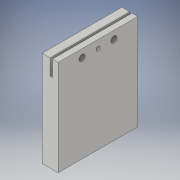
# Autodesk Inventor part: mask holder
Saved by Autodesk Inventor 2017 (Build 210142000, 142)
## iProperties
Created: 2016-12-03
Part Number: mask holder
Material: Generic
Document SubType Name: Modeling
Designer: Darien Morrow
Density: 1 g/cm^3
Appearance: Default
Author: Darien Morrow
Autodesk Inventor part; units mm, degrees
ref_plane "YZ Plane" through (0, 0, 0) normal (1, 0, 0) x (0, 1, 0)
ref_plane "XZ Plane" through (0, 0, 0) normal (0, 1, 0) x (-1, 0, 0)
ref_plane "XY Plane" through (0, 0, 0) normal (0, 0, 1) x (1, 0, 0)
sketch "Sketch1" plane through (0, 0, 0) normal (0, 0, 1) x (1, 0, 0)
  line L0 (-6.35, -38.1) -> (6.35, -38.1)
  line L1 (6.35, -38.1) -> (6.35, 38.1)
  line L2 (6.35, 38.1) -> (-6.35, 38.1)
  line L3 (-6.35, 38.1) -> (-6.35, -38.1)
  line L4 (-6.35, -38.1) -> (6.35, 38.1) construction
  line L5 (6.35, -38.1) -> (-6.35, 38.1) construction
  line L6 (-0.889, 50.8) -> (0.889, 50.8)
  line L7 (0.889, 50.8) -> (0.889, 25.4)
  line L8 (0.889, 25.4) -> (-0.889, 25.4)
  line L9 (-0.889, 25.4) -> (-0.889, 50.8)
  line L10 (-0.889, 50.8) -> (0.889, 25.4) construction
  line L11 (0.889, 50.8) -> (-0.889, 25.4) construction
  point P0 (0, 0)
  point P1 (0, 38.1)
  dimension "d0" = 12.7
  dimension "d1" = 76.2
  dimension "d2" = 1.778
  dimension "d3" = 12.7
  constraints: 24 end point, 5 midpoint, 4 parallel, 2 horizontal, 2 perpendicular
  measures "d0" distance of L2.end L1.end
  measures "d1" distance between parallel lines of L0 L2
  measures "d2" distance of L7.end L8.end
  measures "d3" distance from line of L8 point (0, 38.1)
extrude "Extrusion1" add sketch "Sketch1" along normal blind 63.5 contours L3 L2 L9 L8 L7 L1 L0 | L2 L7 L8 L9
sketch "Sketch2" plane through (0, 0, 0) normal (0, 0, -1) x (-1, 0, 0)
  line L0 (-6.35, 38.1) -> (6.35, 38.1) projected
  line L1 (0, 38.1) -> (-1.778, 38.1)
  line L2 (-1.778, 38.1) -> (-1.778, 25.4)
  line L3 (-1.778, 25.4) -> (0, 25.4)
  line L4 (0, 25.4) -> (0, 38.1)
  point P0 (0, 0)
  dimension "d6" = 1.778
  dimension "d7" = 12.7
  constraints: 8 end point, 2 parallel, 1 horizontal, 1 midpoint, 1 perpendicular
  measures "d6" distance of L3.end L2.end
  measures "d7" distance between parallel lines of L3 L0
extrude "Extrusion2" cut sketch "Sketch2" against normal blind 63.5
sketch "Sketch3" plane through (6.35, -38.1, 0) normal (1, 0, 0) x (0, 0, -1)
  line L0 (0, 76.2) -> (-63.5, 76.2) projected
  line L1 (-63.5, 0) -> (-63.5, 76.2) projected
  point P0 (0, 38.1)
  point P1 (-31.75, 69.85)
  dimension "d10" = 6.35
  dimension "d11" = 31.75
  measures "d10" distance from line of point (-31.75, 69.85) L0
  measures "d11" distance from line of point (-31.75, 69.85) L1
hole "Hole1" at (6.35, 31.75, 31.75) direction (-1, 0, 0) diameter 3.175 end through all
sketch "Sketch4" plane through (6.35, -38.1, 0) normal (1, 0, 0) x (0, 0, -1)
  line L0 (-44.45, 69.8514) -> (-19.05, 69.8514)
  line L1 (0, 0) -> (0, 76.2) projected
  point P0 (0, 38.1)
  dimension "d19" = 25.4
  dimension "d20" = 19.05
  constraints: 2 coincident, 2 end point, 1 horizontal
  measures "d19" distance of L0.start L0.end
  measures "d20" distance from line of L1 L0.end
hole "Hole2" at (6.35, 31.7514, 44.45) at (6.35, 31.7514, 19.05) direction (-1, 0, 0) diameter 4.9784 depth 19.05 tip angle 118 thread size "1/4-20 UNC" class "2B" standard "ANSI Unified Screw Threads"
sketch "Sketch5" plane through (-6.35, -38.1, 0) normal (0, -1, 0) x (1, 0, 0)
  line L0 (6.35, 63.5) -> (6.35, 0) projected
  line L1 (6.35, 57.15) -> (6.35, 6.35)
  dimension "d28" = 50.8
  dimension "d29" = 6.35
  constraints: 2 coincident, 2 end point, 2 point on line
  measures "d28" distance of L1.start L1.end
  measures "d29" distance of L0.start L1.start
hole "Hole3" at (0, -38.1, 57.15) at (0, -38.1, 6.35) direction (0, 1, 0) diameter 5.207 depth 12.7 tip angle 118
sketch "Sketch6" plane through (-6.35, -38.1, 0) normal (0, -1, 0) x (1, 0, 0)
  point P0 (6.35, 0)
sketch "Sketch7" plane through (-6.35, -38.1, 0) normal (0, -1, 0) x (1, 0, 0)
  line L0 (6.35, 63.5) -> (6.35, 0) projected
  line L1 (6.35, 44.45) -> (6.35, 19.05)
  line L2 (0, 63.5) -> (12.7, 63.5) projected
  dimension "d37" = 25.4
  dimension "d38" = 19.05
  constraints: 2 coincident, 2 end point, 2 point on line
  measures "d37" distance of L1.start L1.end
  measures "d38" distance from line of L1.start L2
hole "Hole4" at (0, -38.1, 44.45) at (0, -38.1, 19.05) direction (0, 1, 0) diameter 9.525 depth 5.334 tip angle 118
body "Solid1"
